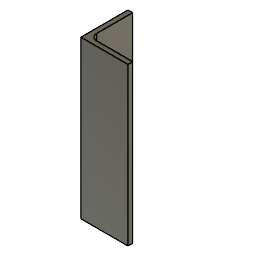
L-30×30×3 (Autodesk Fusion 360 design; units mm, degrees)
Autodesk Fusion 360 part; units mm, degrees
sketch "スケッチ1" plane through (0, 0, 0) normal (0, 0, 1) x (1, 0, 0)
  line L0 (30, 3) -> (7, 3)
  line L1 (0, 0) -> (30, 0)
  line L2 (0, 30) -> (0, 0)
  line L3 (3, 7) -> (3, 30)
  arc A0 (3, 7) -> (7, 3) centre (7, 7) ccw
  line L4 (3, 30) -> (0, 30)
  line L5 (30, 0) -> (30, 3)
extrude "押し出し1" add sketch "スケッチ1" along normal blind 100
